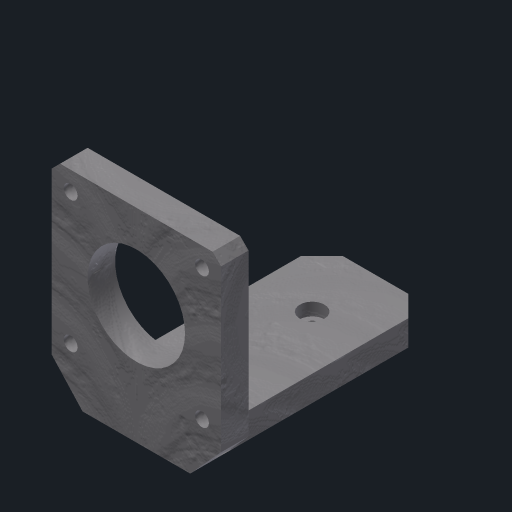
# Autodesk Inventor part: ACOPLE_NEMA_PUERTA
Saved by Autodesk Inventor 2024.3 (Build 283343000, 343)
## iProperties
Created: 2024-06-23
Part Number: ACOPLE_NEMA_PUERTA
Material: Steel, Mild, Welded
Document SubType Name: Modeling
Designer: Niler
Density: 7.85 g/cm^3
Appearance: Weld - Steel Mild
Author: Niler
Autodesk Inventor part; units mm, degrees
ref_plane "YZ Plane" through (0, 0, 0) normal (1, 0, 0) x (0, 1, 0)
ref_plane "XZ Plane" through (0, 0, 0) normal (0, 1, 0) x (-1, 0, 0)
ref_plane "XY Plane" through (0, 0, 0) normal (0, 0, 1) x (1, 0, 0)
sketch "Sketch1" plane through (0, 0, 0) normal (0, 0, 1) x (1, 0, 0)
  line L0 (-20, -20) -> (20, -20)
  line L1 (20, -20) -> (20, 20)
  line L2 (20, 20) -> (-20, 20)
  line L3 (-20, 20) -> (-20, -20)
  line L4 (-20, -20) -> (20, 20) construction
  line L5 (20, -20) -> (-20, 20) construction
  line L6 (-15.5, -15.5) -> (15.5, -15.5) construction
  line L7 (15.5, -15.5) -> (15.5, 15.5) construction
  line L8 (15.5, 15.5) -> (-15.5, 15.5) construction
  line L9 (-15.5, 15.5) -> (-15.5, -15.5) construction
  line L10 (-15.5, -15.5) -> (15.5, 15.5) construction
  line L11 (15.5, -15.5) -> (-15.5, 15.5) construction
  circle A0 centre (-15.5, 15.5) radius 1.65
  circle A1 centre (15.5, 15.5) radius 1.65
  circle A2 centre (15.5, -15.5) radius 1.65
  circle A3 centre (-15.5, -15.5) radius 1.65
  circle A4 centre (0, 0) radius 11.5
  dimension "d0" = 40
  dimension "d1" = 40
  dimension "d2" = 31
  dimension "d3" = 31
  dimension "d4" = 3.3
  dimension "d5" = 23
  constraints: 24 end point, 5 centre point, 5 coincident, 4 midpoint, 4 parallel, 3 equal radius, 2 horizontal, 2 perpendicular
  measures "d0" distance of L2.end L1.end
  measures "d1" distance of L2.end L0.start
  measures "d2" distance of L8.end L7.end
  measures "d3" distance of L7.end L6.end
  measures "d4" diameter of A0
  measures "d5" diameter of A4
extrude "Extrusion1" add sketch "Sketch1" along normal blind 6.5
sketch "Sketch2" plane through (0, 0, 6.5) normal (0, 0, 1) x (1, 0, 0)
  line L0 (-20, -20) -> (20, -20) projected
  line L1 (-20, -20) -> (20, -20) projected
  line L2 (-12.7, -20) -> (12.7, -20)
  line L3 (12.7, -20) -> (12.7, -28)
  line L4 (12.7, -28) -> (-12.7, -28)
  line L5 (-12.7, -28) -> (-12.7, -20)
  line L6 (20, -20) -> (12.7, -28)
  line L7 (-12.7, -28) -> (-20, -20)
  point P0 (0, 0)
  point P1 (0, -28)
  point P2 (0, -20)
  dimension "d8" = 25.4
  dimension "d9" = 8
  constraints: 12 end point, 2 midpoint, 2 parallel, 1 horizontal, 1 perpendicular, 1 point on line, 1 vertical alignment
  measures "d8" distance between parallel lines of L3 L5
  measures "d9" distance of L2.end L3.end
extrude "Extrusion2" add sketch "Sketch2" against normal up to surface (6.5 mm away)
sketch "Sketch3" plane through (0, 0, 0) normal (0, 0, -1) x (-1, 0, 0)
  line L0 (-20, -20) -> (-20, 20) projected
  line L1 (-20, -20) -> (-12.7, -28) projected
  line L2 (-12.7, -28) -> (12.7, -28) projected
  line L3 (12.7, -28) -> (20, -20) projected
  line L4 (20, 20) -> (20, -20) projected
  line L5 (-20, 20) -> (20, 20) projected
  circle A0 centre (15.5, 15.5) radius 1.65 projected
  circle A1 centre (-15.5, 15.5) radius 1.65 projected
  circle A2 centre (-15.5, -15.5) radius 1.65 projected
  circle A3 centre (15.5, -15.5) radius 1.65 projected
  circle A4 centre (0, 0) radius 11.5 projected
  line L6 (-12.7, -28) -> (12.7, -28)
  line L7 (12.7, -28) -> (12.7, -22)
  line L8 (12.7, -22) -> (-12.7, -22)
  line L9 (-12.7, -22) -> (-12.7, -28)
  dimension "d12" = 6
  constraints: 8 end point, 2 parallel, 1 horizontal, 1 perpendicular
  measures "d12" distance between parallel lines of L2 L8
extrude "Extrusion3" add sketch "Sketch3" along normal blind 50 contours L9 L8 L7 L2
fillet "Fillet1" radius 2 1 edges at (0, -22, 0)
fillet "Fillet2" radius 5 4 edges at (12.7, -21, 0) (12.7, -25, 0) (-12.7, -21, 0) (-12.7, -25, 0)
chamfer "Chamfer1" distance 2 angle 45 2 edges at (20, 20, 3.25) (-20, 20, 3.25)
chamfer "Chamfer2" distance 5 angle 45 2 edges at (12.7, -25, -50) (-12.7, -25, -50)
sketch "Sketch4" plane through (-13.7, -22, -2) normal (0, 1, 0) x (1, 0, 0)
  line L0 (1, 43) -> (6, 48) projected
  line L1 (1, 3) -> (1, 43) projected
  arc A0 (0, 0) -> (1, 3) centre (-4, 3) ccw projected
  line L2 (27.4, 0) -> (0, 0) projected
  arc A1 (26.4, 3) -> (27.4, 0) centre (31.4, 3) ccw projected
  line L3 (26.4, 3) -> (26.4, 43) projected
  line L4 (21.4, 48) -> (26.4, 43) projected
  line L5 (6, 48) -> (21.4, 48) projected
  circle A2 centre (13.7, 13) radius 1.65
  circle A3 centre (13.7, 33) radius 1.65
  point P0 (13.7, -2)
  point P1 (13.7, 48)
  dimension "d23" = 3.3
  dimension "d24" = 20
  dimension "d25" = 15
  constraints: 2 centre point, 2 vertical alignment, 1 equal radius, 1 midpoint
  measures "d23" diameter of A2
  measures "d24" distance of A2.centre A3.centre
  measures "d25" distance from line of L5 A3.centre
extrude "Extrusion4" cut sketch "Sketch4" against normal through all contours A2 | A3
sketch "Sketch5" plane through (-13.7, -22, -2) normal (0, 1, 0) x (1, 0, 0)
  circle A0 centre (13.7, 13) radius 1.65 projected
  circle A1 centre (13.7, 33) radius 1.65 projected
  circle A2 centre (13.7, 13) radius 2.9
  circle A3 centre (13.7, 33) radius 2.9
  point P0 (13.7, -2)
  dimension "d28" = 5.8
  constraints: 2 centre point, 2 coincident, 1 equal radius
  measures "d28" diameter of A2
extrude "Extrusion5" cut sketch "Sketch5" against normal blind 3 contours A0 | A1 | A2 | A3
body "Solid1"
